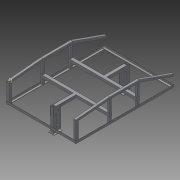
# Autodesk Inventor part: Chassis
Saved by Autodesk Inventor 2015 (Build 190159000, 159)
## iProperties
Created: 2016-02-06
Part Number: Chassis
Material: Generic
Document SubType Name: Modeling
Designer: sethbattis
Density: 1 g/cm^3
Appearance: Default
Author: sethbattis
Autodesk Inventor part; units mm, degrees
ref_plane "YZ Plane" through (0, 0, 0) normal (1, 0, 0) x (0, 1, 0)
ref_plane "XZ Plane" through (0, 0, 0) normal (0, 1, 0) x (-1, 0, 0)
ref_plane "XY Plane" through (0, 0, 0) normal (0, 0, 1) x (1, 0, 0)
sketch "Sketch1" plane through (0, 0, 0) normal (0, 0, 1) x (1, 0, 0)
  line L0 (292.1, 0) -> (292.1, 3.175)
  line L1 (292.1, 3.175) -> (307.975, 3.175)
  line L2 (307.975, 3.175) -> (307.975, 19.05)
  line L3 (307.975, 19.05) -> (311.15, 19.05)
  line L4 (311.15, 19.05) -> (311.15, 0)
  line L5 (311.15, 0) -> (292.1, 0)
  line L6 (-435.61, 0) -> (435.61, 0) construction
  line L7 (0, -3.81) -> (0, 22.86) construction
  line L8 (-292.1, 0) -> (-292.1, 3.175)
  line L9 (-292.1, 3.175) -> (-307.975, 3.175)
  line L10 (-307.975, 3.175) -> (-307.975, 19.05)
  line L11 (-307.975, 19.05) -> (-311.15, 19.05)
  line L12 (-311.15, 19.05) -> (-311.15, 0)
  line L13 (-311.15, 0) -> (-292.1, 0)
  point P0 (0, 0)
  dimension "d4" = 19.05
  dimension "d5" = 3.175
  dimension "d6" = 622.3
  constraints: 24 end point, 9 perpendicular, 6 equal length, 2 collinear, 2 point on line, 2 vertical, 1 other
  measures "d4" distance of L4.end L0.start
  measures "d5" distance of L0.start L0.end
  measures "d6" distance between parallel lines of L4 L12
extrude "Extrusion2" add sketch "Sketch1" along normal blind 876.3
sketch "Sketch2" plane through (-307.975, 19.05, 876.3) normal (1, 0, 0) x (0, 0, -1)
  line L0 (876.3, -15.875) -> (0, -15.875) projected
  line L1 (19.05, -15.875) -> (19.05, -12.7)
  line L2 (19.05, -12.7) -> (3.175, -12.7)
  line L3 (3.175, -12.7) -> (3.175, 3.175)
  line L4 (3.175, 3.175) -> (0, 3.175)
  line L5 (0, 3.175) -> (0, -15.875)
  line L6 (0, -15.875) -> (0, 0) projected
  line L7 (0, -15.875) -> (19.05, -15.875)
  line L8 (0, -15.875) -> (19.05, -15.875)
  line L9 (857.25, -15.875) -> (857.25, -12.7)
  line L10 (857.25, -12.7) -> (873.125, -12.7)
  line L11 (873.125, -12.7) -> (873.125, 3.175)
  line L12 (873.125, 3.175) -> (876.3, 3.175)
  line L13 (876.3, 3.175) -> (876.3, -15.875)
  line L14 (857.25, -15.875) -> (876.3, -15.875)
  line L15 (0, -19.05) -> (0, 0) projected
  point P0 (876.3, -19.05)
  dimension "d9" = 3.175
  dimension "d10" = 19.05
  constraints: 26 end point, 8 perpendicular, 6 equal length, 3 collinear, 2 point on line, 2 vertical
  measures "d9" distance of L1.start L1.end
  measures "d10" distance of L4.end L0.end
extrude "Extrusion3" add sketch "Sketch2" along normal up to surface (615.95 mm away)
sketch "Sketch3" plane through (-307.975, 6.35, 873.125) normal (0, 1, 0) x (1, 0, 0)
  line L0 (615.95, 0) -> (596.9, 0)
  line L1 (596.9, 0) -> (596.9, 23.141)
  line L2 (596.9, 23.141) -> (615.95, 23.141)
  line L3 (615.95, 23.141) -> (615.95, 0)
  line L4 (612.775, 3.175) -> (600.075, 3.175)
  line L5 (600.075, 3.175) -> (600.075, 19.966)
  line L6 (600.075, 19.966) -> (612.775, 19.966)
  line L7 (612.775, 19.966) -> (612.775, 3.175)
  point P0 (307.975, 873.125)
  dimension "d13" = 19.05
  dimension "d14" = 3.175
  dimension "d15" = 3.175
  dimension "d16" = 3.175
  dimension "d17" = 3.175
  constraints: 16 end point, 4 parallel, 2 horizontal, 2 perpendicular
  measures "d13" distance of L1.end L2.end
  measures "d14" distance between parallel lines of L2 L6
  measures "d15" distance between parallel lines of L0 L4
  measures "d16" distance between parallel lines of L3 L7
  measures "d17" distance between parallel lines of L1 L5
extrude "Extrusion4" add sketch "Sketch3" along normal blind 158.75
sketch "Sketch4" plane through (292.1, 3.175, 857.25) normal (0, 1, 0) x (1, 0, 0)
  line L0 (15.875, 285.75) -> (-3.175, 285.75)
  line L1 (-3.175, 285.75) -> (-3.175, 304.8)
  line L2 (-3.175, 304.8) -> (15.875, 304.8)
  line L3 (15.875, 304.8) -> (15.875, 285.75)
  line L4 (-600.075, -19.05) -> (15.875, -19.05) projected
  line L5 (15.875, 552.45) -> (-3.175, 552.45)
  line L6 (-3.175, 552.45) -> (-3.175, 533.4)
  line L7 (-3.175, 533.4) -> (15.875, 533.4)
  line L8 (15.875, 533.4) -> (15.875, 552.45)
  line L9 (12.7, 549.275) -> (0, 549.275)
  line L10 (0, 549.275) -> (0, 536.575)
  line L11 (0, 536.575) -> (12.7, 536.575)
  line L12 (12.7, 536.575) -> (12.7, 549.275)
  line L13 (12.7, 301.625) -> (0, 301.625)
  line L14 (0, 301.625) -> (0, 288.925)
  line L15 (0, 288.925) -> (12.7, 288.925)
  line L16 (12.7, 288.925) -> (12.7, 301.625)
  line L17 (15.875, 854.075) -> (15.875, 7.266) projected
  line L18 (-600.075, 857.25) -> (15.875, 857.25) projected
  point P0 (-292.1, 857.25)
  dimension "d24" = 19.05
  dimension "d25" = 19.05
  dimension "d26" = 304.8
  dimension "d27" = 19.05
  dimension "d28" = 19.05
  dimension "d31" = 3.175
  dimension "d32" = 3.175
  dimension "d33" = 3.175
  dimension "d34" = 3.175
  dimension "d35" = 3.175
  dimension "d36" = 3.175
  dimension "d78" = 304.8
  constraints: 32 end point, 8 parallel, 4 horizontal, 4 perpendicular, 2 equal length, 1 collinear
  measures "d24" distance of L1.end L2.end
  measures "d25" distance of L0.end L1.end
  measures "d26" distance between parallel lines of L0 L4
  measures "d27" distance of L7.end L6.end
  measures "d28" distance of L6.end L5.end
  measures "d31" distance between parallel lines of L5 L9
  measures "d32" distance between parallel lines of L7 L11
  measures "d33" distance between parallel lines of L8 L12
  measures "d34" distance between parallel lines of L6 L10
  measures "d35" distance between parallel lines of L3 L16
  measures "d36" distance between parallel lines of L2 L13
  measures "d78" distance between parallel lines of L18 L5
extrude "Extrusion5" add sketch "Sketch4" along normal blind 187.325
ref_plane "Work Plane1" through (0, 0, 0) normal (1, 0, 0) x (0, 0, -1)
mirror "Mirror1" about plane through (0, 0, 0) normal (1, 0, 0) of "Extrusion4", "Extrusion5"
sketch "Sketch5" plane through (-307.975, 19.05, 323.85) normal (-1, 0, 0) x (0, 0, 1)
  line L0 (-22.225, 63.5) -> (3.175, 63.5)
  line L1 (3.175, 63.5) -> (3.175, 38.1)
  line L2 (3.175, 38.1) -> (-22.225, 38.1)
  line L3 (-22.225, 38.1) -> (-22.225, 63.5)
  line L4 (-19.05, 60.325) -> (0, 60.325)
  line L5 (0, 60.325) -> (0, 41.275)
  line L6 (0, 41.275) -> (-19.05, 41.275)
  line L7 (-19.05, 41.275) -> (-19.05, 60.325)
  line L8 (-19.05, 0) -> (-19.05, 171.45) projected
  line L9 (-323.85, -19.05) -> (552.45, -19.05) projected
  line L10 (225.425, 63.5) -> (250.825, 63.5)
  line L11 (250.825, 63.5) -> (250.825, 38.1)
  line L12 (250.825, 38.1) -> (225.425, 38.1)
  line L13 (225.425, 38.1) -> (225.425, 63.5)
  line L14 (228.6, 60.325) -> (247.65, 60.325)
  line L15 (247.65, 60.325) -> (247.65, 41.275)
  line L16 (247.65, 41.275) -> (228.6, 41.275)
  line L17 (228.6, 41.275) -> (228.6, 60.325)
  line L18 (247.65, 0) -> (247.65, 171.45) projected
  point P0 (247.65, -15.875)
  dimension "d39" = 25.4
  dimension "d40" = 25.4
  dimension "d41" = 3.175
  dimension "d42" = 3.175
  dimension "d43" = 19.05
  dimension "d44" = 19.05
  dimension "d45" = 57.15
  dimension "d46" = 3.175
  dimension "d47" = 3.175
  constraints: 32 end point, 8 parallel, 4 equal length, 4 horizontal, 4 perpendicular, 3 collinear
  measures "d39" distance of L1.end L2.end
  measures "d40" distance of L0.end L1.end
  measures "d41" distance between parallel lines of L0 L4
  measures "d42" distance between parallel lines of L1 L5
  measures "d43" distance of L4.start L4.end
  measures "d44" distance of L4.end L5.end
  measures "d45" distance between parallel lines of L2 L9
  measures "d46" distance between parallel lines of L10 L14
  measures "d47" distance between parallel lines of L11 L15
extrude "Extrusion6" add sketch "Sketch5" against normal up to surface (615.95 mm away) contours L0 L8 L7 L2 L3 | L0 L1 L2 L8 L6 L5 L4 | L10 L18 L14 L17 L16 L12 L13 | L10 L11 L12 L18 L15
sketch "Sketch6" plane through (-307.975, 57.15, 301.625) normal (0, 0, -1) x (-1, 0, 0)
  line L0 (0, 0) -> (-615.95, 0) projected
  line L1 (-320.675, 25.4) -> (-295.275, 25.4)
  line L2 (-295.275, 25.4) -> (-295.275, 0)
  line L3 (-295.275, 0) -> (-320.675, 0)
  line L4 (-320.675, 0) -> (-320.675, 25.4)
  line L5 (-19.05, 22.225) -> (-596.9, 22.225) projected
  line L6 (-19.05, 3.175) -> (-596.9, 3.175) projected
  line L7 (-317.5, 22.225) -> (-298.45, 22.225)
  line L8 (-298.45, 22.225) -> (-298.45, 3.175)
  line L9 (-298.45, 3.175) -> (-317.5, 3.175)
  line L10 (-317.5, 3.175) -> (-317.5, 22.225)
  line L11 (-307.975, -95.25) -> (-307.975, 171.45) projected
  line L12 (0, 25.4) -> (-615.95, 25.4) projected
  point P0 (-307.975, -57.15)
  constraints: 16 end point, 4 parallel, 4 perpendicular, 3 point on line, 2 horizontal, 1 collinear, 2 other
extrude "Extrusion7" add sketch "Sketch6" along normal blind 177.8 contours L0 L11 L6 L2 | L0 L4 L6 L11 | L6 L8 L5 L2 | L5 L11 L1 L2 | L4 L5 L10 L6 | L5 L4 L1 L11
sketch "Sketch7" plane through (-307.975, 82.55, 327.025) normal (0, 1, 0) x (1, 0, 0)
  line L0 (320.675, 203.2) -> (295.275, 203.2)
  line L1 (295.275, 203.2) -> (295.275, 228.6)
  line L2 (295.275, 228.6) -> (320.675, 228.6)
  line L3 (320.675, 228.6) -> (320.675, 203.2)
  line L4 (295.275, 203.2) -> (320.675, 203.2) projected
  line L5 (295.275, 25.4) -> (295.275, 203.2) projected
  line L6 (317.5, 206.375) -> (298.45, 206.375)
  line L7 (298.45, 206.375) -> (298.45, 225.425)
  line L8 (298.45, 225.425) -> (317.5, 225.425)
  line L9 (317.5, 225.425) -> (317.5, 206.375)
  point P0 (307.975, 327.025)
  dimension "d53" = 3.175
  dimension "d54" = 3.175
  dimension "d55" = 3.175
  dimension "d56" = 3.175
  constraints: 16 end point, 4 parallel, 3 perpendicular, 2 horizontal, 1 collinear
  measures "d53" distance between parallel lines of L3 L9
  measures "d54" distance between parallel lines of L0 L6
  measures "d55" distance between parallel lines of L1 L7
  measures "d56" distance between parallel lines of L2 L8
extrude "Extrusion8" add sketch "Sketch7" against normal blind 203.2
sketch "Sketch8" plane through (-12.7, 57.15, 123.825) normal (0, 0, 1) x (1, 0, 0)
  line L0 (12.7, 195.58) -> (12.7, -240.03) projected
  line L1 (0, -177.8) -> (25.4, -177.8) projected
  line L2 (11.1125, -6.35) -> (14.2875, -6.35)
  line L3 (14.2875, -6.35) -> (14.2875, -177.8)
  line L4 (14.2875, -177.8) -> (11.1125, -177.8)
  line L5 (11.1125, -177.8) -> (11.1125, -6.35)
  point P0 (12.7, -57.15)
  dimension "d59" = 3.175
  dimension "d60" = 171.45
  constraints: 8 end point, 2 parallel, 1 horizontal, 1 perpendicular, 1 point on line, 1 other
  measures "d59" distance of L2.start L2.end
  measures "d60" distance of L2.end L3.end
extrude "Extrusion9" add sketch "Sketch8" along normal blind 50.8
sketch "Sketch9" plane through (-307.975, -120.65, 327.025) normal (0, -1, 0) x (1, 0, 0)
  line L0 (307.975, 724.535) -> (307.975, -502.285) projected
  line L1 (282.575, -161.925) -> (333.375, -161.925)
  line L2 (333.375, -161.925) -> (333.375, -234.95)
  line L3 (333.375, -234.95) -> (282.575, -234.95)
  line L4 (282.575, -234.95) -> (282.575, -161.925)
  line L5 (295.275, -228.6) -> (320.675, -228.6) projected
  point P0 (307.975, -327.025)
  dimension "d63" = 50.8
  dimension "d64" = 6.35
  dimension "d65" = 73.025
  constraints: 8 end point, 2 parallel, 1 horizontal, 1 perpendicular, 1 other
  measures "d63" distance of L2.end L3.end
  measures "d64" distance between parallel lines of L5 L3
  measures "d65" distance of L3.end L1.start
extrude "Extrusion10" add sketch "Sketch9" along normal blind 3.175
sketch "Sketch14" plane through (1.5875, -120.65, 174.625) normal (1, 0, 0) x (0, 0, -1)
  line L0 (25.4, 318.5116) -> (25.4, -2.4611)
  line L1 (0.11, 38.1) -> (94.3477, 38.1)
  line L2 (0.11, 139.7) -> (94.3477, 139.7)
  line L3 (9.525, 0) -> (82.55, 0) projected
  line L4 (0, 0) -> (0, 171.45) projected
  line L5 (50.8, 177.8) -> (50.8, 0) projected
  line L6 (174.625, 139.7) -> (-701.675, 139.7) projected
  point P0 (174.625, 120.65)
  point P1 (25.4, 139.7)
  point P2 (25.4, 38.1)
  dimension "d79" = 101.6
  dimension "d80" = 38.1
  dimension "d81" = 25.4
  constraints: 6 end point, 4 point on line, 2 horizontal, 1 vertical
  measures "d79" distance between parallel lines of L1 L2
  measures "d80" distance between parallel lines of L3 L1
  measures "d81" distance between parallel lines of L0 L4
hole "Hole1" at (1.5875, 19.05, 149.225) at (1.5875, -82.55, 149.225) direction (-1, 0, 0) diameter 19.05 end up to face face through (-1.5875, -6.35, 154.5167) facing (-1, 0, 0)
ref_plane "Work Plane2" through (-307.975, 57.15, 438.15) normal (0, 0, 1) x (1, 0, 0)
mirror "Mirror2" about plane through (-307.975, 57.15, 438.15) normal (0, 0, 1) of "Extrusion7", "Extrusion8", "Extrusion9", "Extrusion10", "Hole1"
sketch "Sketch21" plane through (12.7, -120.65, 777.875) normal (1, 0, 0) x (0, 0, -1)
  line L0 (203.2, 203.2) -> (0, 203.2) projected
  line L1 (76.2, 203.2) -> (0, 127)
  line L2 (0, 127) -> (0, 203.2)
  line L3 (3.175, 203.2) -> (3.175, 0) projected
  line L4 (0, 203.2) -> (76.2, 203.2)
  line L5 (76.2, 0) -> (76.2, 171.45) projected
  point P0 (777.875, 120.65)
  constraints: 6 end point, 2 perpendicular, 2 point on line, 1 parallel
extrude "Extrusion14" add sketch "Sketch21" along normal blind 3.175 draft 0.125
mirror "Mirror5" about plane through (0, 0, 0) normal (1, 0, 0) of "Extrusion14"
sketch "Sketch10" plane through (-288.925, 190.5, 304.8) normal (0, 0, -1) x (-1, 0, 0)
  line L0 (-597.1227, 0) -> (-577.85, 0)
  line L1 (-577.85, 0) -> (-577.85, 19.05)
  line L2 (-577.85, 19.05) -> (-597.1227, 19.05)
  line L3 (-597.1227, 19.05) -> (-597.1227, 0)
  line L4 (-577.85, -107.95) -> (-577.85, 0) projected
  line L5 (-596.9, 0) -> (-577.85, 0) projected
  line L6 (-593.725, 15.875) -> (-581.025, 15.875)
  line L7 (-581.025, 15.875) -> (-581.025, 3.175)
  line L8 (-581.025, 3.175) -> (-593.725, 3.175)
  line L9 (-593.725, 3.175) -> (-593.725, 15.875)
  line L10 (-581.025, -107.95) -> (-581.025, 0) projected
  line L11 (-593.725, -107.95) -> (-593.725, 0) projected
  point P0 (-288.925, -190.5)
  dimension "d68" = 3.175
  dimension "d69" = 3.175
  constraints: 16 end point, 4 collinear, 4 parallel, 4 perpendicular, 2 horizontal
  measures "d68" distance between parallel lines of L0 L8
  measures "d69" distance between parallel lines of L1 L7
extrude "Extrusion11" add sketch "Sketch10" against normal up to surface (266.7 mm away)
sketch "Sketch12" plane through (307.975, 19.05, 849.984) normal (1, 0, 0) x (0, 0, -1)
  line L0 (0, 146.05) -> (278.484, 171.45)
  line L1 (0, 146.05) -> (-2.1019, 169.0953)
  line L2 (-23.141, 146.05) -> (0, 146.05) projected
  point P0 (849.984, -19.05)
  constraints: 4 end point, 1 equal length, 1 perpendicular
ref_plane "Work Plane3" through (307.975, 165.1, 849.984) normal (0, 0.0908311, -0.9958663) x (-1, 0, 0)
sketch "Sketch13" plane through (307.975, 165.1, 849.984) normal (0, 0.0908311, -0.9958663) x (-1, 0, 0)
  line L0 (0, 19.05) -> (19.05, 19.05)
  line L1 (19.05, 19.05) -> (19.05, 0)
  line L2 (19.05, 0) -> (0, 0)
  line L3 (0, 0) -> (0, 19.05)
  line L4 (0, 0) -> (0, 23.141) projected
  line L5 (19.05, -140.1825) -> (19.05, 2.1019) projected
  line L6 (0, 0) -> (19.05, 0) projected
  line L7 (15.875, 15.875) -> (3.175, 15.875)
  line L8 (3.175, 15.875) -> (3.175, 3.175)
  line L9 (3.175, 3.175) -> (15.875, 3.175)
  line L10 (15.875, 3.175) -> (15.875, 15.875)
  point P0 (307.975, -241.6225)
  dimension "d72" = 19.05
  dimension "d73" = 12.7
  dimension "d74" = 3.175
  dimension "d75" = 3.175
  constraints: 16 end point, 4 parallel, 4 perpendicular, 2 collinear, 2 horizontal
  measures "d72" distance of L0.start L0.end
  measures "d73" distance of L7.start L7.end
  measures "d74" distance between parallel lines of L0 L7
  measures "d75" distance between parallel lines of L1 L10
extrude "Extrusion12" add sketch "Sketch13" against normal up to surface starts on plane at (288.925, 3.175, 571.5) facing (0, 0, 1) surface through (288.925, 6.35, 873.125) normal (0, 0, 1)
mirror "Mirror3" about plane through (0, 0, 0) normal (1, 0, 0) of "Extrusion11", "Extrusion12"
sketch "Sketch18" plane through (308.1977, 190.5, 304.8) normal (1, 0, 0) x (0, 0, -1)
  line L0 (0, 19.05) -> (0, 0)
  line L1 (0, 19.05) -> (0, 0) projected
  line L2 (0, 0) -> (285.75, -101.6)
  line L3 (285.75, -101.6) -> (285.75, -187.325)
  line L4 (304.8, -190.5) -> (-571.5, -190.5) projected
  line L5 (0, 0) -> (6.3819, 17.9492)
  dimension "d94" = 88.9
  constraints: 8 end point, 1 collinear, 1 equal length, 1 perpendicular, 1 vertical
  measures "d94" distance from line of L2.end L4
sketch "Sketch19" plane through (288.925, 82.55, 304.8) normal (-1, 0, 0) x (0, 0, 1)
  point P0 (-304.8, -82.55)
  point P1 (0, 107.95)
ref_plane "Work Plane6" through (308.1977, 208.4492, 298.4181) normal (0, -0.3350097, -0.9422147) x (0, -0.9422147, 0.3350097)
sketch "Sketch20" plane through (308.1977, 208.4492, 298.4181) normal (0, -0.3350097, -0.9422147) x (0, -0.9422147, 0.3350097)
  line L0 (0, 0) -> (19.05, 0)
  line L1 (19.05, 0) -> (19.05, 19.05)
  line L2 (19.05, 19.05) -> (0, 19.05)
  line L3 (0, 19.05) -> (0, 0)
  line L4 (3.175, 3.175) -> (16.0977, 3.175)
  line L5 (16.0977, 3.175) -> (16.0977, 16.0977)
  line L6 (16.0977, 16.0977) -> (3.175, 16.0977)
  line L7 (3.175, 16.0977) -> (3.175, 3.175)
  line L8 (1.1008, 19.2727) -> (1.1008, 0) projected
  line L9 (4.0923, 3.3977) -> (4.0923, 16.0977) projected
  line L10 (4.0923, 16.0977) -> (93.4394, 16.0977) projected
  point P0 (96.431, 308.1977)
  dimension "d95" = 3.175
  dimension "d96" = 3.175
  dimension "d99" = 19.05
  constraints: 16 end point, 4 parallel, 4 perpendicular, 2 horizontal, 1 coincident, 1 collinear
  measures "d95" distance between parallel lines of L0 L4
  measures "d96" distance between parallel lines of L3 L7
  measures "d99" distance of L2.end L0.start
extrude "Extrusion13" add sketch "Sketch20" along normal up to surface starts on plane at (307.975, 3.175, 304.8) facing (0, 0, -1) surface through (304.9323, 6.2177, 0) normal (0, 0, 1)
mirror "Mirror4" about plane through (0, 0, 0) normal (1, 0, 0) of "Extrusion13"
mirror "Mirror6" about plane through (-307.975, 57.15, 438.15) normal (0, 0, 1) of "Extrusion14", "Mirror5"
ref_plane "Work Plane4" through (-307.975, 165.1, 849.984) normal (0, -0.0908311, 0.9958663) x (1, 0, 0)
body "Solid2"
